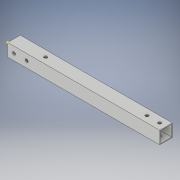
# Autodesk Inventor part: Vertical
Saved by Autodesk Inventor 2017 (Build 210142000, 142)
## iProperties
Created: 2018-07-12
Part Number: Vertical
Material: Generic
Document SubType Name: Modeling
Designer: sinner
Density: 1 g/cm^3
Appearance: Default
Author: sinner
Autodesk Inventor part; units mm, degrees
ref_plane "YZ Plane" through (0, 0, 0) normal (1, 0, 0) x (0, 1, 0)
ref_plane "XZ Plane" through (0, 0, 0) normal (0, 1, 0) x (-1, 0, 0)
ref_plane "XY Plane" through (0, 0, 0) normal (0, 0, 1) x (1, 0, 0)
sketch "Sketch1" plane through (0, 0, 0) normal (1, 0, 0) x (0, 1, 0)
  line L0 (0, 0) -> (25.4, 0)
  line L1 (25.4, 0) -> (25.4, -25.4)
  line L2 (25.4, -25.4) -> (0, -25.4)
  line L3 (0, -25.4) -> (0, 0)
  line L4 (23.8125, -23.8125) -> (23.8125, -1.5875)
  line L5 (23.8125, -1.5875) -> (1.5875, -1.5875)
  line L6 (1.5875, -1.5875) -> (1.5875, -23.8125)
  line L7 (1.5875, -23.8125) -> (23.8125, -23.8125)
  dimension "d0" = 25.4
  dimension "d1" = 25.4
  dimension "d2" = 1.5875
  constraints: 16 end point, 4 parallel, 2 perpendicular, 1 horizontal, 3 other
  measures "d0" distance of L1.end L2.end
  measures "d1" distance of L0.end L1.end
  measures "d2" distance between parallel lines of L1 L4
extrude "Extrusion1" add sketch "Sketch1" along normal blind 304.8
sketch "Sketch2" plane through (0, 25.4, 0) normal (0, 1, 0) x (1, 0, 0)
  line L0 (304.8, 1.5875) -> (304.8, 23.8125) projected
  line L1 (304.8, 12.7) -> (279.4, 12.7) construction
  circle A0 centre (292.1, 12.7) radius 3.175
  line L2 (304.8, 25.4) -> (304.8, 0) projected
  circle A1 centre (266.7, 12.7) radius 3.175
  circle A2 centre (63.5, 12.7) radius 3.175
  line L3 (0, 0) -> (0, 25.4) projected
  dimension "d5" = 6.35
  dimension "d6" = 12.7
  dimension "d9" = 38.1
  dimension "d15" = 63.5
  constraints: 3 centre point, 2 end point, 2 equal radius, 2 midpoint, 2 point on line, 1 horizontal
  measures "d5" diameter of A0
  measures "d6" distance from line of L2 A0.centre
  measures "d9" distance from line of A1.centre L0
  measures "d15" distance from line of L3 A2.centre
extrude "Extrusion2" cut sketch "Sketch2" against normal blind 25.4
sketch "Sketch3" plane through (0, 0, 0) normal (0, 0, 1) x (1, 0, 0)
  line L0 (0, 0) -> (0, 25.4) projected
  line L1 (0, 12.7) -> (67.237, 12.7) construction
  circle A0 centre (12.7, 12.7) radius 3.175
  circle A1 centre (38.1, 12.7) radius 3.175
  dimension "d10" = 6.35
  dimension "d11" = 12.7
  dimension "d12" = 38.1
  constraints: 2 centre point, 2 end point, 2 point on line, 1 equal radius, 1 horizontal, 1 midpoint
  measures "d10" diameter of A1
  measures "d11" distance from line of L0 A0.centre
  measures "d12" distance from line of L0 A1.centre
extrude "Extrusion3" cut sketch "Sketch3" against normal blind 25.4
sketch "Sketch4" plane through (0, 25.4, 0) normal (0, 1, 0) x (1, 0, 0)
  point P0 (0, 0)
body "Solid1"
